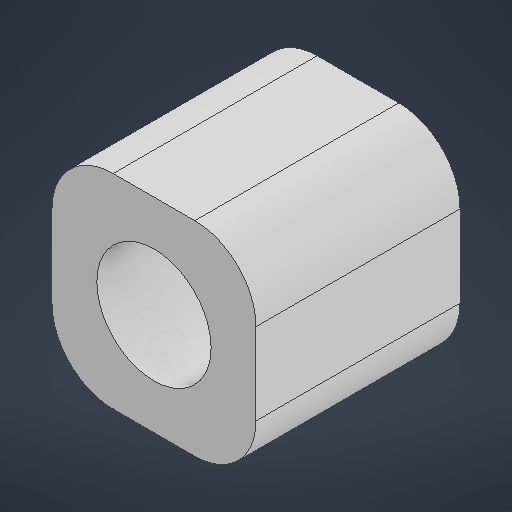
# Autodesk Inventor part: ReyenedorTornillo3M
Saved by Autodesk Inventor 2026.2 (Build 302298010, 298A)
## iProperties
Created: 2026-04-22
Part Number: ReyenedorTornillo3M
Material: Genérico
Document SubType Name: Modeling
Designer: Jose Carlos
Density: 1 g/cm^3
Appearance: Valor por defecto
Author: Jose Carlos
Autodesk Inventor part; units mm, degrees
ref_plane "YZ Plane" through (0, 0, 0) normal (1, 0, 0) x (0, 1, 0)
ref_plane "XZ Plane" through (0, 0, 0) normal (0, 1, 0) x (-1, 0, 0)
ref_plane "Plano de trabajo1" through (0, 0, 0) normal (0, 0, 1) x (1, 0, 0)
sketch "Boceto1" plane through (0, 0, 0) normal (0, 0, 1) x (1, 0, 0)
  circle A0 centre (-10, -5) radius 1.5 construction
  line L0 (-11, -2.5) -> (-9, -2.5)
  line L1 (-7.5, -4) -> (-7.5, -6)
  line L2 (-9, -7.5) -> (-11, -7.5)
  line L3 (-12.5, -6) -> (-12.5, -4)
  line L4 (-12.5, -2.5) -> (-7.5, -7.5) construction
  line L5 (-7.5, -2.5) -> (-12.5, -7.5) construction
  arc A1 (-9, -7.5) -> (-7.5, -6) centre (-9, -6) ccw
  arc A2 (-12.5, -6) -> (-11, -7.5) centre (-11, -6) ccw
  arc A3 (-7.5, -4) -> (-9, -2.5) centre (-9, -4) ccw
  arc A4 (-11, -2.5) -> (-12.5, -4) centre (-11, -4) ccw
  circle A5 centre (-10, -5) radius 1.4
  point P0 (0, 0)
  dimension "d0" = 5
  dimension "d1" = 5
  dimension "d2" = 1.5
  dimension "d5" = 0.1
  constraints: 12 end point, 8 point on circle, 8 point on line, 8 tangent, 5 centre point, 3 equal radius, 2 midpoint, 2 parallel, 1 coincident, 1 horizontal, 1 perpendicular
  measures "d0" distance of L4.end L5.end
  measures "d1" distance of L5.start L4.end
  measures "d2" radius of A1
  measures "d5" radial gap between concentric circles of A0 A5
extrude "Extrusión1" add sketch "Boceto1" along normal blind 5
